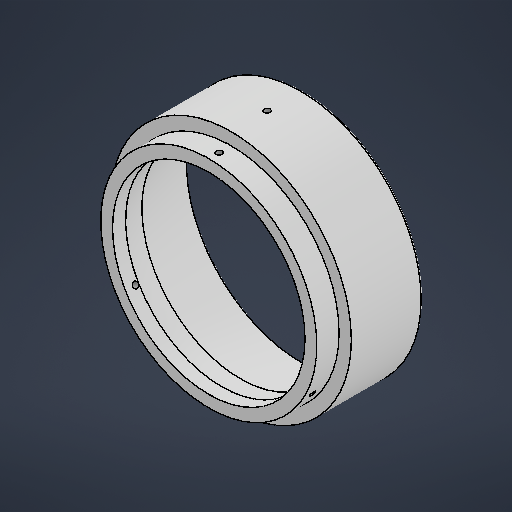
# Autodesk Inventor part: Tail
Saved by Autodesk Inventor 2026.1 (Build 301233000, 233)
## iProperties
Created: 2025-09-27
Part Number: Tail
Material: Generic
Document SubType Name: Modeling
Designer: 1char
Mass: 64.5255 g
Surface Area: 262.951 cm^2
Volume: 64.5255 cm^3
Density: 1 g/cm^3
Appearance: Default
Author: 1char
Autodesk Inventor part; units mm, degrees
ref_plane "YZ Plane" through (0, 0, 0) normal (1, 0, 0) x (0, 1, 0)
ref_plane "XZ Plane" through (0, 0, 0) normal (0, 1, 0) x (-1, 0, 0)
ref_plane "XY Plane" through (0, 0, 0) normal (0, 0, 1) x (1, 0, 0)
sketch "Sketch1" plane through (0, 0, 0) normal (0, 0, 1) x (1, 0, 0)
  circle A0 centre (0, 0) radius 40
  circle A1 centre (0, 0) radius 50
  dimension "d0" = 80
  dimension "d1" = 100
  constraints: 2 centre point, 2 coincident
  measures "d0" diameter of A0
  measures "d1" diameter of A1
extrude "Extrusion1" add sketch "Sketch1" against normal blind 30
sketch "Sketch2" plane through (0, 0, 0) normal (0, 0, 1) x (1, 0, 0)
  circle A0 centre (0, 0) radius 44.9
  circle A1 centre (0, 0) radius 40 projected
  dimension "d4" = 89.8
  constraints: 1 centre point, 1 coincident
  measures "d4" diameter of A0
extrude "Extrusion2" add sketch "Sketch2" along normal blind 9.25
sketch "Sketch3" plane through (0, 0, 0) normal (0, 1, 0) x (-1, 0, 0)
  point P0 (0, 0)
  point P1 (0, 5)
  dimension "d7" = 5
  constraints: 1 vertical alignment
  measures "d7" distance of point (0, 0) point (0, 5)
hole "Hole1" at (0, 0, 5) direction (0, 1, 0) diameter 2.459 end through all thread size "M3x0.5" class "6H" standard "ISO Metric profile"
pattern_circular "Circular Pattern1" count 3 over 360 about axis through (0, 0, -10) along (0, 0, 1) of "Hole1"
sketch "Sketch4" plane through (0, 0, 0) normal (0, 1, 0) x (-1, 0, 0)
  point P0 (0, -15)
  point P1 (0, 0)
  dimension "d23" = 15
  constraints: 1 vertical alignment
  measures "d23" distance of point (0, -15) point (0, 0)
hole "Hole2" at (0, 0, -15) direction (0, 1, 0) diameter 2.459 end through all counterbore diameter 6.5 counterbore depth 3.4 thread size "M3x0.5" class "6H" standard "ANSI Metric M Profile"
chamfer "Chamfer1" distance 8 angle 75 1 edges at (-40, 0, -30)
fillet "Fillet1" radius 30 1 edges at (-40, 0, -0.1436)
fillet "Fillet2" radius 1 2 edges at (-48, 0, -30) (-50, 0, -30)
body "Solid1"
